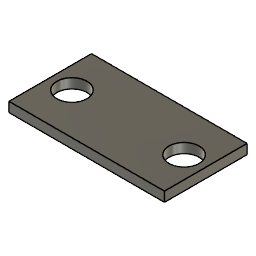
bottom (Autodesk Fusion 360 design; units mm, degrees)
Autodesk Fusion 360 part; units mm, degrees
sketch "Sketch1" plane through (0, 0, 0) normal (0, 0, 1) x (1, 0, 0)
  line L0 (0, 0) -> (111, 0)
  line L1 (111, 0) -> (111, -59)
  line L2 (111, -59) -> (0, -59)
  line L3 (0, -59) -> (0, 0)
  line L4 (95.5, 0) -> (95.5, -59)
  line L5 (15.5, -59) -> (15.5, 0)
  line L6 (0, -29.5) -> (111, -29.5)
  circle A0 centre (95.5, -29.5) radius 10.75
  circle A1 centre (15.5, -29.5) radius 10.75
  dimension "d1" = 111
  dimension "d2" = 59
  dimension "d3" = 15.5
  dimension "d4" = 15.5
  dimension "d5" = 29.5
  dimension "d6" = 21.5
  dimension "d7" = 21.5
  constraint coincident L0.start L3.end
  constraint horizontal L0
  constraint perpendicular L0 L1
  constraint perpendicular L1 L2
  constraint perpendicular L0 L3
  constraint midpoint L4 A0.centre
  constraint midpoint L5 A1.centre
  constraint coincident L0 L4.start
  constraint coincident L2 L4.end
  constraint coincident L2 L5.start
  constraint coincident L0 L5.end
  constraint vertical L2.end L6.start
  constraint vertical L0.end L6.end
  measures "d1" distance of L0.start L0.end
  measures "d2" distance of L0.end L1.end
  measures "d6" diameter of A0
  measures "d7" diameter of A1
extrude "Extrude1" add sketch "Sketch1" along normal blind 7 contours L0 L3 L5 L6 A1 | L0 L4 L5 L6 A0 A1 | L2 L3 L5 L6 A1 | L0 L1 L4 L6 A0 | L2 L4 L5 L6 A0 A1 | L1 L2 L4 L6 A0
